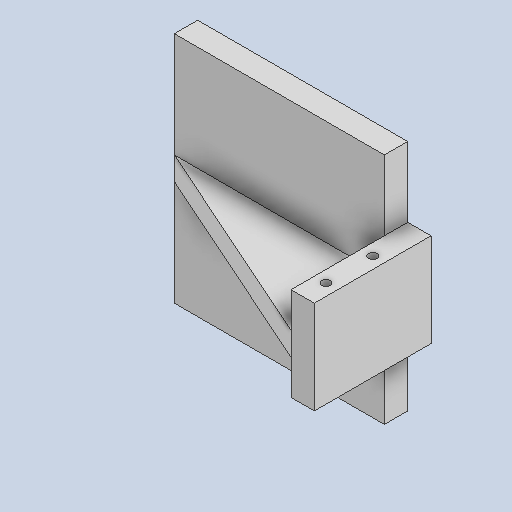
# Autodesk Inventor part: Finger
Saved by Autodesk Inventor 2023 (Build 270158000, 158)
## iProperties
Created: 2023-01-25
Part Number: Finger
Material: Generic
Document SubType Name: Modeling
Designer: Gabriel - T3 CAD
Density: 1 g/cm^3
Appearance: Default
Mass: 260.383 g
Surface Area: 499.728 cm^2
Volume: 260.383 cm^3
Author: Gabriel - T3 CAD
Autodesk Inventor part; units mm, degrees
ref_plane "YZ Plane" through (0, 0, 0) normal (1, 0, 0) x (0, 1, 0)
ref_plane "XZ Plane" through (0, 0, 0) normal (0, 1, 0) x (-1, 0, 0)
ref_plane "XY Plane" through (0, 0, 0) normal (0, 0, 1) x (1, 0, 0)
sketch "Sketch1" plane through (0, 0, 0) normal (0, 1, 0) x (-1, 0, 0)
  line L0 (0, 0) -> (12.7, 0)
  line L1 (12.7, 0) -> (12.7, 63.5)
  line L2 (12.7, 63.5) -> (0, 63.5)
  line L3 (0, 63.5) -> (0, 0)
  line L4 (0, 0) -> (127, 0)
  line L5 (127, 0) -> (127, 12.7)
  line L6 (127, 12.7) -> (0, 12.7)
  line L7 (0, 12.7) -> (0, 0)
  circle A0 centre (6.35, 50.8) radius 2.3813
  circle A1 centre (6.35, 25.4) radius 2.3813
  line L8 (12.7, 63.5) -> (127, 12.7)
  point P0 (12.7, 12.7)
  dimension "d0" = 12.7
  dimension "d1" = 63.5
  dimension "d2" = 127
  dimension "d3" = 12.7
  dimension "d4" = 25.4
  dimension "d5" = 6.35
  dimension "d6" = 6.35
  dimension "d7" = 12.7
  dimension "d8" = 4.7625
  dimension "d9" = 4.7625
  constraints: 18 end point, 4 parallel, 2 centre point, 2 horizontal, 2 perpendicular
  measures "d0" distance of L2.end L1.end
  measures "d1" distance of L1.end L0.end
  measures "d2" distance of L6.end L5.end
  measures "d3" distance of L5.end L4.end
  measures "d4" distance of A1.centre A0.centre
  measures "d5" distance from line of L3 A0.centre
  measures "d6" distance from line of L3 A1.centre
  measures "d7" distance from line of L2 A0.centre
  measures "d8" diameter of A0
  measures "d9" diameter of A1
extrude "Extrusion1" add sketch "Sketch1" along normal mid plane 50.8 contours L3 L2 L1 L6
extrude "Extrusion2" add sketch "Sketch1" along normal mid plane 127 contours L1 L6 L5 L4
extrude "Extrusion3" add sketch "Sketch1" along normal mid plane 12.7 contours L1 L8 L6
sketch "Sketch2" plane through (0, -25.4, 63.5) normal (1, 0, 0) x (0, 0, -1)
  line L0 (0, 50.8) -> (50.8, 50.8) projected
  line L1 (50.8, 50.8) -> (63.5, 50.8)
  line L2 (63.5, 50.8) -> (63.5, 63.5)
  line L3 (63.5, 63.5) -> (50.8, 63.5)
  line L4 (50.8, 63.5) -> (50.8, 50.8)
  line L5 (50.8, 0) -> (0, 0) projected
  line L6 (50.8, 0) -> (63.5, 0)
  line L7 (63.5, 0) -> (63.5, -12.7)
  line L8 (63.5, -12.7) -> (50.8, -12.7)
  line L9 (50.8, -12.7) -> (50.8, 0)
  line L10 (63.5, -38.1) -> (63.5, 88.9) projected
  line L11 (63.5, 0) -> (63.5, 50.8)
  line L12 (50.8, 0) -> (50.8, 50.8) projected
  line L13 (50.8, 50.8) -> (50.8, 0)
  point P0 (63.5, 25.4)
  dimension "d16" = 12.7
  dimension "d17" = 12.7
  dimension "d18" = 12.7
  dimension "d19" = 12.7
  constraints: 20 end point, 5 equal length, 2 horizontal, 2 perpendicular
  measures "d16" distance of L3.end L2.end
  measures "d17" distance of L2.end L1.end
  measures "d18" distance of L7.end L8.end
  measures "d19" distance of L6.end L7.end
extrude "Extrusion4" add sketch "Sketch2" against normal blind 12.7 contours L1 L10 L6 L12
body "Solid1"
